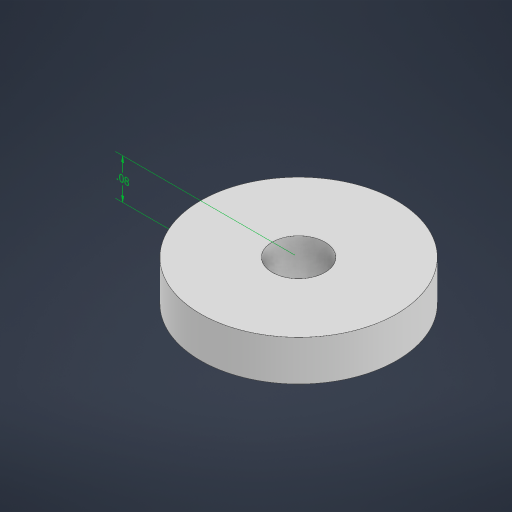
# Autodesk Inventor part: ArmSpacerMini
Saved by Autodesk Inventor 2024.2 (Build 282272000, 272)
## iProperties
Created: 2024-01-19
Part Number: ArmSpacerMini
Material: Generic
Document SubType Name: Modeling
Designer: ctam0
Density: 1 g/cm^3
Appearance: Default
Author: ctam0
Autodesk Inventor part; units mm, degrees
ref_plane "YZ Plane" through (0, 0, 0) normal (1, 0, 0) x (0, 1, 0)
ref_plane "XZ Plane" through (0, 0, 0) normal (0, 1, 0) x (-1, 0, 0)
ref_plane "XY Plane" through (0, 0, 0) normal (0, 0, 1) x (1, 0, 0)
sketch "Sketch1" plane through (0, 0, 0) normal (0, 1, 0) x (-1, 0, 0)
  circle A0 centre (0, 0) radius 4.9276
  circle A1 centre (0, 0) radius 1.3208
  dimension "d0" = 9.8552
  dimension "d1" = 2.6416
  constraints: 2 centre point, 2 coincident
  measures "d0" diameter of A0
  measures "d1" diameter of A1
extrude "Extrusion1" add sketch "Sketch1" along normal blind 2.032
body "Solid1"
